Autodesk Inventor part; units mm, degrees
(part 3 of 4)
sketch "Эскиз9" plane through (0, 0, 5) normal (0, 0, 1) x (1, 0, 0)
  circle A0 centre (1.2104, 5.1192) radius 2.5 projected
  circle A1 centre (1.2104, 5.1192) radius 12.2678
  line L0 (44.0249, 7.1187) -> (57, -5.9715) projected
  line L1 (57, -5.9715) -> (57, 20.778) projected
  line L2 (53, 20.778) -> (57, 20.778) projected
  line L3 (25.3405, 9.161) -> (53, 20.778) projected
  arc A2 (16.1963, 14.3431) -> (25.3405, 9.161) centre (40.8164, 47.1281) ccw projected
  arc A3 (16.1963, 14.3431) -> (-11.1891, 14.3431) centre (2.5036, -3.8906) ccw projected
  line L4 (-11.1891, 14.3431) -> (-11.0924, 14.1698) projected
  line L5 (-11.0924, 14.1698) -> (-10.8798, 13.8428) projected
  line L6 (-10.8798, 13.8428) -> (-10.6476, 13.5415) projected
  line L7 (-10.6476, 13.5415) -> (-10.3902, 13.2744) projected
  line L8 (-10.3902, 13.2744) -> (-10.0964, 13.0589) projected
  line L9 (-10.0964, 13.0589) -> (-9.8198, 12.8188) projected
  line L10 (-9.8198, 12.8188) -> (-9.6918, 12.6838) projected
  line L11 (-9.6918, 12.6838) -> (-9.5723, 12.5363) projected
  line L12 (-9.5723, 12.5363) -> (-9.4633, 12.3731) projected
  line L13 (-9.4633, 12.3731) -> (-9.3681, 12.1883) projected
  line L14 (-9.3681, 12.1883) -> (-9.3278, 12.0845) projected
  line L15 (-9.3278, 12.0845) -> (-9.2943, 11.9695) projected
  line L16 (-9.2943, 11.9695) -> (-9.2712, 11.8376) projected
  line L17 (-9.2712, 11.8376) -> (-9.2668, 11.6743) projected
  line L18 (-9.2668, 11.6743) -> (-9.3696, 11.329) projected
  line L19 (-9.3696, 11.329) -> (-9.7265, 10.6764) projected
  line L20 (-9.7265, 10.6764) -> (-10.0432, 10.0032) projected
  line L21 (-10.0432, 10.0032) -> (-10.2615, 9.7167) projected
  line L22 (-10.2615, 9.7167) -> (-10.3959, 9.6239) projected
  line L23 (-10.3959, 9.6239) -> (-10.5161, 9.5649) projected
  line L24 (-10.5161, 9.5649) -> (-10.6287, 9.5241) projected
  line L25 (-10.6287, 9.5241) -> (-10.7364, 9.4955) projected
  line L26 (-10.7364, 9.4955) -> (-10.9417, 9.4634) projected
  line L27 (-10.9417, 9.4634) -> (-11.1379, 9.4552) projected
  line L28 (-11.1379, 9.4552) -> (-11.3274, 9.4648) projected
  line L29 (-11.3274, 9.4648) -> (-11.5119, 9.4885) projected
  line L30 (-11.5119, 9.4885) -> (-11.8689, 9.5704) projected
  line L31 (-11.8689, 9.5704) -> (-12.2162, 9.6807) projected
  line L32 (-12.2162, 9.6807) -> (-12.5837, 9.731) projected
  line L33 (-12.5837, 9.731) -> (-12.964, 9.741) projected
  line L34 (-12.964, 9.741) -> (-13.3534, 9.7199) projected
  line L35 (-13.3534, 9.7199) -> (-13.7498, 9.6714) projected
  line L36 (-13.7498, 9.6714) -> (-14.1519, 9.5976) projected
  line L37 (-14.1519, 9.5976) -> (-14.5586, 9.4998) projected
  line L38 (-14.5586, 9.4998) -> (-14.9687, 9.3787) projected
  line L39 (-14.9687, 9.3787) -> (-15.3815, 9.2349) projected
  line L40 (-15.3815, 9.2349) -> (-15.796, 9.069) projected
  line L41 (-15.796, 9.069) -> (-16.1075, 8.9301) projected
  line L42 (-16.1075, 8.9301) -> (-16.4414, 6.8067) projected
  line L43 (-16.4414, 6.8067) -> (-16.1875, 6.579) projected
  line L44 (-16.1875, 6.579) -> (-15.8439, 6.2938) projected
  line L45 (-15.8439, 6.2938) -> (-15.4952, 6.0303) projected
  line L46 (-15.4952, 6.0303) -> (-15.142, 5.7892) projected
  line L47 (-15.142, 5.7892) -> (-14.785, 5.5713) projected
  line L48 (-14.785, 5.5713) -> (-14.425, 5.3776) projected
  line L49 (-14.425, 5.3776) -> (-14.0625, 5.2099) projected
  line L50 (-14.0625, 5.2099) -> (-13.6984, 5.0703) projected
  line L51 (-13.6984, 5.0703) -> (-13.3334, 4.963) projected
  line L52 (-13.3334, 4.963) -> (-12.9682, 4.8982) projected
  line L53 (-12.9682, 4.8982) -> (-12.6038, 4.8965) projected
  line L54 (-12.6038, 4.8965) -> (-12.2389, 4.8649) projected
  line L55 (-12.2389, 4.8649) -> (-12.056, 4.8309) projected
  line L56 (-12.056, 4.8309) -> (-11.8727, 4.7818) projected
  line L57 (-11.8727, 4.7818) -> (-11.6885, 4.7139) projected
  line L58 (-11.6885, 4.7139) -> (-11.5029, 4.6203) projected
  line L59 (-11.5029, 4.6203) -> (-11.4093, 4.56) projected
  line L60 (-11.4093, 4.56) -> (-11.3146, 4.4866) projected
  line L61 (-11.3146, 4.4866) -> (-11.2183, 4.3936) projected
  line L62 (-11.2183, 4.3936) -> (-11.1188, 4.264) projected
  line L63 (-11.1188, 4.264) -> (-10.999, 3.9243) projected
  line L64 (-10.999, 3.9243) -> (-10.9042, 3.1865) projected
  line L65 (-10.9042, 3.1865) -> (-10.7647, 2.4558) projected
  line L66 (-10.7647, 2.4558) -> (-10.7729, 2.0956) projected
  line L67 (-10.7729, 2.0956) -> (-10.8272, 1.9416) projected
  line L68 (-10.8272, 1.9416) -> (-10.8897, 1.8232) projected
  line L69 (-10.8897, 1.8232) -> (-10.9568, 1.724) projected
  line L70 (-10.9568, 1.724) -> (-11.0271, 1.6375) projected
  line L71 (-11.0271, 1.6375) -> (-11.1743, 1.4909) projected
  line L72 (-11.1743, 1.4909) -> (-11.3282, 1.369) projected
  line L73 (-11.3282, 1.369) -> (-11.4872, 1.2653) projected
  line L74 (-11.4872, 1.2653) -> (-11.6504, 1.1761) projected
  line L75 (-11.6504, 1.1761) -> (-11.9874, 1.0325) projected
  line L76 (-11.9874, 1.0325) -> (-12.3332, 0.9175) projected
  line L77 (-12.3332, 0.9175) -> (-12.66, 0.7423) projected
  line L78 (-12.66, 0.7423) -> (-12.9736, 0.5268) projected
  line L79 (-12.9736, 0.5268) -> (-13.2762, 0.2808) projected
  line L80 (-13.2762, 0.2808) -> (-13.5684, 0.0086) projected
  line L81 (-13.5684, 0.0086) -> (-13.8504, -0.2874) projected
  line L82 (-13.8504, -0.2874) -> (-14.1218, -0.6056) projected
  line L83 (-14.1218, -0.6056) -> (-14.3824, -0.9447) projected
  line L84 (-14.3824, -0.9447) -> (-14.6319, -1.3036) projected
  line L85 (-14.6319, -1.3036) -> (-14.8697, -1.6815) projected
  line L86 (-14.8697, -1.6815) -> (-15.0401, -1.9769) projected
  line L87 (-15.0401, -1.9769) -> (-14.0621, -3.891) projected
  line L88 (-14.0621, -3.891) -> (-13.7228, -3.9261) projected
  line L89 (-13.7228, -3.9261) -> (-13.2773, -3.9548) projected
  line L90 (-13.2773, -3.9548) -> (-12.8403, -3.963) projected
  line L91 (-12.8403, -3.963) -> (-12.4128, -3.9505) projected
  line L92 (-12.4128, -3.9505) -> (-11.9959, -3.917) projected
  line L93 (-11.9959, -3.917) -> (-11.5908, -3.862) projected
  line L94 (-11.5908, -3.862) -> (-11.199, -3.7847) projected
  line L95 (-11.199, -3.7847) -> (-10.8224, -3.6836) projected
  line L96 (-10.8224, -3.6836) -> (-10.464, -3.5558) projected
  line L97 (-10.464, -3.5558) -> (-10.1304, -3.3936) projected
  line L98 (-10.1304, -3.3936) -> (-9.8347, -3.1808) projected
  line L99 (-9.8347, -3.1808) -> (-9.5209, -2.9918) projected
  line L100 (-9.5209, -2.9918) -> (-9.353, -2.9118) projected
  line L101 (-9.353, -2.9118) -> (-9.1758, -2.8438) projected
  line L102 (-9.1758, -2.8438) -> (-8.9868, -2.7905) projected
  line L103 (-8.9868, -2.7905) -> (-8.7817, -2.7571) projected
  line L104 (-8.7817, -2.7571) -> (-8.6705, -2.7509) projected
  line L105 (-8.6705, -2.7509) -> (-8.5508, -2.7546) projected
  line L106 (-8.5508, -2.7546) -> (-8.4182, -2.7733) projected
  line L107 (-8.4182, -2.7733) -> (-8.2615, -2.8196) projected
  line L108 (-8.2615, -2.8196) -> (-7.9649, -3.024) projected
  line L109 (-7.9649, -3.024) -> (-7.4545, -3.5652) projected
  line L110 (-7.4545, -3.5652) -> (-6.9122, -4.0744) projected
  line L111 (-6.9122, -4.0744) -> (-6.7071, -4.3705) projected
  line L112 (-6.7071, -4.3705) -> (-6.6604, -4.5271) projected
  line L113 (-6.6604, -4.5271) -> (-6.6415, -4.6596) projected
  line L114 (-6.6415, -4.6596) -> (-6.6374, -4.7793) projected
  line L115 (-6.6374, -4.7793) -> (-6.6435, -4.8906) projected
  line L116 (-6.6435, -4.8906) -> (-6.6764, -5.0958) projected
  line L117 (-6.6764, -5.0958) -> (-6.7292, -5.2848) projected
  line L118 (-6.7292, -5.2848) -> (-6.7969, -5.4622) projected
  line L119 (-6.7969, -5.4622) -> (-6.8765, -5.6303) projected
  line L120 (-6.8765, -5.6303) -> (-7.0647, -5.9445) projected
  line L121 (-7.0647, -5.9445) -> (-7.2769, -6.2407) projected
  line L122 (-7.2769, -6.2407) -> (-7.4384, -6.5746) projected
  line L123 (-7.4384, -6.5746) -> (-7.5654, -6.9333) projected
  line L124 (-7.5654, -6.9333) -> (-7.6656, -7.3102) projected
  line L125 (-7.6656, -7.3102) -> (-7.742, -7.7022) projected
  line L126 (-7.742, -7.7022) -> (-7.7961, -8.1074) projected
  line L127 (-7.7961, -8.1074) -> (-7.8287, -8.5243) projected
  line L128 (-7.8287, -8.5243) -> (-7.8403, -8.9518) projected
  line L129 (-7.8403, -8.9518) -> (-7.8311, -9.3888) projected
  line L130 (-7.8311, -9.3888) -> (-7.8013, -9.8343) projected
  line L131 (-7.8013, -9.8343) -> (-7.7656, -10.1735) projected
  line L132 (-7.7656, -10.1735) -> (-5.8492, -11.1472) projected
  line L133 (-5.8492, -11.1472) -> (-5.5542, -10.9761) projected
  line L134 (-5.5542, -10.9761) -> (-5.1768, -10.7375) projected
  line L135 (-5.1768, -10.7375) -> (-4.8185, -10.4872) projected
  line L136 (-4.8185, -10.4872) -> (-4.48, -10.2258) projected
  line L137 (-4.48, -10.2258) -> (-4.1624, -9.9537) projected
  line L138 (-4.1624, -9.9537) -> (-3.867, -9.6711) projected
  line L139 (-3.867, -9.6711) -> (-3.5955, -9.3782) projected
  line L140 (-3.5955, -9.3782) -> (-3.3502, -9.0751) projected
  line L141 (-3.3502, -9.0751) -> (-3.1354, -8.7611) projected
  line L142 (-3.1354, -8.7611) -> (-2.9609, -8.4338) projected
  line L143 (-2.9609, -8.4338) -> (-2.8467, -8.0877) projected
  line L144 (-2.8467, -8.0877) -> (-2.7039, -7.7505) projected
  line L145 (-2.7039, -7.7505) -> (-2.615, -7.5871) projected
  line L146 (-2.615, -7.5871) -> (-2.5117, -7.4278) projected
  line L147 (-2.5117, -7.4278) -> (-2.3901, -7.2737) projected
  line L148 (-2.3901, -7.2737) -> (-2.2438, -7.1261) projected
  line L149 (-2.2438, -7.1261) -> (-2.1575, -7.0556) projected
  line L150 (-2.1575, -7.0556) -> (-2.0585, -6.9883) projected
  line L151 (-2.0585, -6.9883) -> (-1.9402, -6.9255) projected
  line L152 (-1.9402, -6.9255) -> (-1.7863, -6.8709) projected
  line L153 (-1.7863, -6.8709) -> (-1.4262, -6.8619) projected
  line L154 (-1.4262, -6.8619) -> (-0.6951, -6.9997) projected
  line L155 (-0.6951, -6.9997) -> (0.0429, -7.0929) projected
  line L156 (0.0429, -7.0929) -> (0.3829, -7.2119) projected
  line L157 (0.3829, -7.2119) -> (0.5127, -7.3112) projected
  line L158 (0.5127, -7.3112) -> (0.6059, -7.4072) projected
  line L159 (0.6059, -7.4072) -> (0.6795, -7.5017) projected
  line L160 (0.6795, -7.5017) -> (0.74, -7.5953) projected
  line L161 (0.74, -7.5953) -> (0.834, -7.7806) projected
  line L162 (0.834, -7.7806) -> (0.9024, -7.9646) projected
  line L163 (0.9024, -7.9646) -> (0.9519, -8.1479) projected
  line L164 (0.9519, -8.1479) -> (0.9863, -8.3307) projected
  line L165 (0.9863, -8.3307) -> (1.0187, -8.6955) projected
  line L166 (1.0187, -8.6955) -> (1.0212, -9.0599) projected
  line L167 (1.0212, -9.0599) -> (1.0869, -9.4249) projected
  line L168 (1.0869, -9.4249) -> (1.1949, -9.7897) projected
  line L169 (1.1949, -9.7897) -> (1.3353, -10.1535) projected
  line L170 (1.3353, -10.1535) -> (1.5039, -10.5156) projected
  line L171 (1.5039, -10.5156) -> (1.6983, -10.8752) projected
  line L172 (1.6983, -10.8752) -> (1.9171, -11.2317) projected
  line L173 (1.9171, -11.2317) -> (2.159, -11.5843) projected
  line L174 (2.159, -11.5843) -> (2.4233, -11.9325) projected
  line L175 (2.4233, -11.9325) -> (2.7092, -12.2754) projected
  line L176 (2.7092, -12.2754) -> (2.9375, -12.5288) projected
  line L177 (2.9375, -12.5288) -> (5.0602, -12.1901) projected
  line L178 (5.0602, -12.1901) -> (5.1983, -11.8783) projected
  line L179 (5.1983, -11.8783) -> (5.3633, -11.4634) projected
  line L180 (5.3633, -11.4634) -> (5.5062, -11.0504) projected
  line L181 (5.5062, -11.0504) -> (5.6263, -10.6399) projected
  line L182 (5.6263, -10.6399) -> (5.7233, -10.2331) projected
  line L183 (5.7233, -10.2331) -> (5.7962, -9.8308) projected
  line L184 (5.7962, -9.8308) -> (5.8437, -9.4343) projected
  line L185 (5.8437, -9.4343) -> (5.864, -9.0449) projected
  line L186 (5.864, -9.0449) -> (5.8532, -8.6645) projected
  line L187 (5.8532, -8.6645) -> (5.802, -8.2972) projected
  line L188 (5.802, -8.2972) -> (5.691, -7.9502) projected
  line L189 (5.691, -7.9502) -> (5.6083, -7.5933) projected
  line L190 (5.6083, -7.5933) -> (5.5841, -7.4089) projected
  line L191 (5.5841, -7.4089) -> (5.5741, -7.2193) projected
  line L192 (5.5741, -7.2193) -> (5.5818, -7.0232) projected
  line L193 (5.5818, -7.0232) -> (5.6135, -6.8178) projected
  line L194 (5.6135, -6.8178) -> (5.6419, -6.7101) projected
  line L195 (5.6419, -6.7101) -> (5.6824, -6.5974) projected
  line L196 (5.6824, -6.5974) -> (5.7412, -6.4771) projected
  line L197 (5.7412, -6.4771) -> (5.8336, -6.3424) projected
  line L198 (5.8336, -6.3424) -> (6.1197, -6.1235) projected
  line L199 (6.1197, -6.1235) -> (6.7921, -5.8052) projected
  line L200 (6.7921, -5.8052) -> (7.444, -5.4468) projected
  line L201 (7.444, -5.4468) -> (7.789, -5.3433) projected
  line L202 (7.789, -5.3433) -> (7.9523, -5.3473) projected
  line L203 (7.9523, -5.3473) -> (8.0842, -5.3702) projected
  line L204 (8.0842, -5.3702) -> (25.3405, 4.0009) projected
  line L205 (40.9018, 10.5367) -> (25.3405, 4.0009) projected
  line L206 (40.9018, 10.5367) -> (44.0249, 7.1187) projected
  circle A4 centre (1.2104, 5.1192) radius 2.5 projected
  circle A5 centre (4.7663, 12.2855) radius 1.6 projected
  circle A6 centre (-5.9559, 8.675) radius 1.6 projected
  circle A7 centre (-2.3455, -2.0471) radius 1.6 projected
  circle A8 centre (8.3767, 1.5633) radius 1.6 projected
  point P0 (0, 0)
  point P1 (-10.9042, 3.1865)
  constraints: 1 coincident, 3 other
extrude "Выдавливание9" cut sketch "Эскиз9" against normal through all contours A1 L18 L17 L16 L15 L14 L13 L12 L11 L10 L9 L8 L7 L6 L5 L4 A3 A2 L3 L2 L1 L0 L206 L205 L204 L203 L202 L201
sketch "Эскиз18" plane through (0, 0, 5) normal (0, 0, 1) x (1, 0, 0)
  arc A0 (-3.5282, 16.5591) -> (-4.3322, 16.1919) centre (1.2104, 5.1192) ccw
  arc A1 (-6.5592, 14.7607) -> (-7.2273, 14.1819) centre (1.2104, 5.1192) ccw
  arc A2 (-8.9608, 12.1812) -> (-9.4387, 11.4376) centre (1.2104, 5.1192) ccw
  arc A3 (-10.7875, 8.1814) -> (-13.7875, 7.8251) centre (-10.997, -2.8603) ccw
  arc A4 (-13.7875, 7.8251) -> (-13.9423, 6.7483) centre (1.2104, 5.1192) ccw
  arc A5 (-13.9423, 6.7483) -> (-11.1642, 5.5611) centre (-8.2544, 16.2146) ccw
  arc A6 (-11.1642, 5.5611) -> (-11.1642, 4.6772) centre (1.2104, 5.1192) ccw
  arc A7 (-11.1642, 4.6772) -> (-13.9423, 3.4901) centre (-8.2544, -5.9763) ccw
  arc A8 (-13.9423, 3.4901) -> (-13.7875, 2.4133) centre (1.2104, 5.1192) ccw
  arc A9 (-13.7875, 2.4133) -> (-10.7875, 2.0569) centre (-10.997, 13.0986) ccw
  arc A10 (-10.7875, 2.0569) -> (-10.5384, 1.2088) centre (1.2104, 5.1192) ccw
  arc A11 (-10.5384, 1.2088) -> (-12.8695, -0.7129) centre (-4.7451, -8.1934) ccw
  arc A12 (-12.8695, -0.7129) -> (-12.4176, -1.7025) centre (1.2104, 5.1192) ccw
  arc A13 (-12.4176, -1.7025) -> (-9.4387, -1.1992) centre (-12.7506, 9.3362) ccw
  arc A14 (-9.4387, -1.1992) -> (-8.9608, -1.9429) centre (1.2104, 5.1192) ccw
  arc A15 (-8.9608, -1.9429) -> (-10.6561, -4.4435) centre (-0.7533, -9.332) ccw
  arc A16 (-10.6561, -4.4435) -> (-9.9437, -5.2656) centre (1.2104, 5.1192) ccw
  arc A17 (-9.9437, -5.2656) -> (-7.2273, -3.9435) centre (-13.3732, 5.2321) ccw
  arc A18 (-7.2273, -3.9435) -> (-6.5592, -4.5224) centre (1.2104, 5.1192) ccw
  arc A19 (-6.5592, -4.5224) -> (-7.4813, -7.3993) centre (3.3977, -9.2999) ccw
  arc A20 (-7.4813, -7.3993) -> (-6.5661, -7.9874) centre (1.2104, 5.1192) ccw
  arc A21 (-6.5661, -7.9874) -> (-4.3322, -5.9536) centre (-12.8142, 1.1189) ccw
  arc A22 (-4.3322, -5.9536) -> (-3.5282, -6.3208) centre (1.2104, 5.1192) ccw
  arc A23 (-3.5282, -6.3208) -> (-3.6024, -9.3409) centre (7.3714, -8.0996) ccw
  arc A24 (-3.6024, -9.3409) -> (-2.5586, -9.6474) centre (1.2104, 5.1192) ccw
  arc A25 (-2.5586, -9.6474) -> (-0.9882, -7.0666) centre (-11.1191, -2.6703) ccw
  arc A26 (-0.9882, -7.0666) -> (-0.1132, -7.1924) centre (1.2104, 5.1192) ccw
  arc A27 (-0.1132, -7.1924) -> (0.6664, -10.1111) centre (10.846, -5.8284) ccw
  arc A28 (0.6664, -10.1111) -> (1.7543, -10.1111) centre (1.2104, 5.1192) ccw
  arc A29 (1.7543, -10.1111) -> (2.534, -7.1924) centre (-8.4252, -5.8284) ccw
  arc A30 (2.534, -7.1924) -> (3.409, -7.0666) centre (1.2104, 5.1192) ccw
  arc A31 (3.409, -7.0666) -> (4.9793, -9.6474) centre (13.5399, -2.6703) ccw
  arc A32 (4.9793, -9.6474) -> (6.0232, -9.3409) centre (1.2104, 5.1192) ccw
  arc A33 (6.0232, -9.3409) -> (5.949, -6.3208) centre (-4.9506, -8.0996) ccw
  arc A34 (5.949, -6.3208) -> (6.753, -5.9536) centre (1.2104, 5.1192) ccw
  arc A35 (8.98, -4.5224) -> (9.6481, -3.9435) centre (1.2104, 5.1192) ccw
  arc A36 (11.3816, -1.9429) -> (11.8595, -1.1992) centre (1.2104, 5.1192) ccw
  arc A37 (12.9592, 1.2088) -> (13.2083, 2.0569) centre (1.2104, 5.1192) ccw
  arc A38 (13.585, 4.6772) -> (13.585, 5.5611) centre (1.2104, 5.1192) ccw
  arc A39 (13.2083, 8.1814) -> (12.9592, 9.0296) centre (1.2104, 5.1192) ccw
  arc A40 (11.8595, 11.4376) -> (11.3816, 12.1812) centre (1.2104, 5.1192) ccw
  arc A41 (9.6481, 14.1819) -> (8.98, 14.7607) centre (1.2104, 5.1192) ccw
  arc A42 (6.753, 16.1919) -> (5.949, 16.5591) centre (1.2104, 5.1192) ccw
  arc A43 (3.409, 17.3049) -> (2.534, 17.4307) centre (1.2104, 5.1192) ccw
  arc A44 (-0.1132, 17.4307) -> (-0.9882, 17.3049) centre (1.2104, 5.1192) ccw
  circle A45 centre (1.2104, 5.1192) radius 2.5 projected
  circle A46 centre (-2.3455, -2.0471) radius 1.6 projected
  circle A47 centre (-5.9559, 8.675) radius 1.6 projected
  circle A48 centre (8.3767, 1.5633) radius 1.6 projected
  circle A49 centre (4.7663, 12.2855) radius 1.6 projected
  circle A50 centre (1.2104, 5.1192) radius 12.3825
  line L0 (-10.7875, 8.1814) -> (1.2104, 5.1192)
  point P0 (0, 0)
  point P1 (1.2104, 5.1192)
  point P2 (6.753, -5.9536)
  point P3 (8.98, -4.5224)
  point P4 (9.6481, -3.9435)
  point P5 (11.3816, -1.9429)
  point P6 (11.8595, -1.1992)
  point P7 (13.2083, 2.0569)
  point P8 (13.585, 4.6772)
  point P9 (13.585, 5.5611)
  point P10 (13.2083, 8.1814)
  point P11 (12.9592, 9.0296)
  point P12 (11.8595, 11.4376)
  point P13 (11.3816, 12.1812)
  point P14 (8.98, 14.7607)
  point P15 (5.949, 16.5591)
  point P16 (3.409, 17.3049)
  point P17 (2.534, 17.4307)
  point P18 (-0.1132, 17.4307)
  point P19 (-0.9882, 17.3049)
  point P20 (-3.5282, 16.5591)
  point P21 (-4.3322, 16.1919)
  point P22 (-6.5592, 14.7607)
  point P23 (-7.2273, 14.1819)
  point P24 (-9.4387, 11.4376)
  point P25 (3.409, -7.0666)
  point P26 (2.534, -7.1924)
  point P27 (-0.1132, -7.1924)
  point P28 (-0.9882, -7.0666)
  point P29 (-3.5282, -6.3208)
  point P30 (-4.3322, -5.9536)
  point P31 (-6.5592, -4.5224)
  point P32 (-7.2273, -3.9435)
  point P33 (-8.9608, -1.9429)
  point P34 (-9.4387, -1.1992)
  point P35 (-10.5384, 1.2088)
  point P36 (-10.7875, 2.0569)
  point P37 (-11.1642, 4.6772)
  point P38 (-11.1642, 5.5611)
  constraints: 90 point on circle, 45 centre point, 2 end point, 1 coincident, 4 other
sketch "Эскиз19" plane through (0, 0, 5) normal (0, 0, 1) x (1, 0, 0)
  arc A0 (7.444, -5.4468) -> (-9.3696, 11.329) centre (1.2104, 5.1192) ccw projected
  line L0 (-9.3696, 11.329) -> (-9.7265, 10.6764) projected
  line L1 (-9.7265, 10.6764) -> (-10.0432, 10.0032) projected
  line L2 (-10.0432, 10.0032) -> (-10.2615, 9.7167) projected
  line L3 (-10.2615, 9.7167) -> (-10.3959, 9.6239) projected
  line L4 (-10.3959, 9.6239) -> (-10.5161, 9.5649) projected
  line L5 (-10.5161, 9.5649) -> (-10.6287, 9.5241) projected
  line L6 (-10.6287, 9.5241) -> (-10.7364, 9.4955) projected
  line L7 (-10.7364, 9.4955) -> (-10.9417, 9.4634) projected
  line L8 (-10.9417, 9.4634) -> (-11.1379, 9.4552) projected
  line L9 (-11.1379, 9.4552) -> (-11.3274, 9.4648) projected
  line L10 (-11.3274, 9.4648) -> (-11.5119, 9.4885) projected
  line L11 (-11.5119, 9.4885) -> (-11.8689, 9.5704) projected
  line L12 (-11.8689, 9.5704) -> (-12.2162, 9.6807) projected
  line L13 (-12.2162, 9.6807) -> (-12.5837, 9.731) projected
  line L14 (-12.5837, 9.731) -> (-12.964, 9.741) projected
  line L15 (-12.964, 9.741) -> (-13.3534, 9.7199) projected
  line L16 (-13.3534, 9.7199) -> (-13.7498, 9.6714) projected
  line L17 (-13.7498, 9.6714) -> (-14.1519, 9.5976) projected
  line L18 (-14.1519, 9.5976) -> (-14.5586, 9.4998) projected
  line L19 (-14.5586, 9.4998) -> (-14.9687, 9.3787) projected
  line L20 (-14.9687, 9.3787) -> (-15.3815, 9.2349) projected
  line L21 (-15.3815, 9.2349) -> (-15.796, 9.069) projected
  line L22 (-15.796, 9.069) -> (-16.1075, 8.9301) projected
  line L23 (-16.1075, 8.9301) -> (-16.4414, 6.8067) projected
  line L24 (-16.4414, 6.8067) -> (-16.1875, 6.579) projected
  line L25 (-16.1875, 6.579) -> (-15.8439, 6.2938) projected
  line L26 (-15.8439, 6.2938) -> (-15.4952, 6.0303) projected
  line L27 (-15.4952, 6.0303) -> (-15.142, 5.7892) projected
  line L28 (-15.142, 5.7892) -> (-14.785, 5.5713) projected
  line L29 (-14.785, 5.5713) -> (-14.425, 5.3776) projected
  line L30 (-14.425, 5.3776) -> (-14.0625, 5.2099) projected
  line L31 (-14.0625, 5.2099) -> (-13.6984, 5.0703) projected
  line L32 (-13.6984, 5.0703) -> (-13.3334, 4.963) projected
  line L33 (-13.3334, 4.963) -> (-12.9682, 4.8982) projected
  line L34 (-12.9682, 4.8982) -> (-12.6038, 4.8965) projected
  line L35 (-12.6038, 4.8965) -> (-12.2389, 4.8649) projected
  line L36 (-12.2389, 4.8649) -> (-12.056, 4.8309) projected
  line L37 (-12.056, 4.8309) -> (-11.8727, 4.7818) projected
  line L38 (-11.8727, 4.7818) -> (-11.6885, 4.7139) projected
  line L39 (-11.6885, 4.7139) -> (-11.5029, 4.6203) projected
  line L40 (-11.5029, 4.6203) -> (-11.4093, 4.56) projected
  line L41 (-11.4093, 4.56) -> (-11.3146, 4.4866) projected
  line L42 (-11.3146, 4.4866) -> (-11.2183, 4.3936) projected
  line L43 (-11.2183, 4.3936) -> (-11.1188, 4.264) projected
  line L44 (-11.1188, 4.264) -> (-10.999, 3.9243) projected
  line L45 (-10.999, 3.9243) -> (-10.9042, 3.1865) projected
  line L46 (-10.9042, 3.1865) -> (-10.7647, 2.4558) projected
  line L47 (-10.7647, 2.4558) -> (-10.7729, 2.0956) projected
  line L48 (-10.7729, 2.0956) -> (-10.8272, 1.9416) projected
  line L49 (-10.8272, 1.9416) -> (-10.8897, 1.8232) projected
  line L50 (-10.8897, 1.8232) -> (-10.9568, 1.724) projected
  line L51 (-10.9568, 1.724) -> (-11.0271, 1.6375) projected
  line L52 (-11.0271, 1.6375) -> (-11.1743, 1.4909) projected
  line L53 (-11.1743, 1.4909) -> (-11.3282, 1.369) projected
  line L54 (-11.3282, 1.369) -> (-11.4872, 1.2653) projected
  line L55 (-11.4872, 1.2653) -> (-11.6504, 1.1761) projected
  line L56 (-11.6504, 1.1761) -> (-11.9874, 1.0325) projected
  line L57 (-11.9874, 1.0325) -> (-12.3332, 0.9175) projected
  line L58 (-12.3332, 0.9175) -> (-12.66, 0.7423) projected
  line L59 (-12.66, 0.7423) -> (-12.9736, 0.5268) projected
  line L60 (-12.9736, 0.5268) -> (-13.2762, 0.2808) projected
  line L61 (-13.2762, 0.2808) -> (-13.5684, 0.0086) projected
  line L62 (-13.5684, 0.0086) -> (-13.8504, -0.2874) projected
  line L63 (-13.8504, -0.2874) -> (-14.1218, -0.6056) projected
  line L64 (-14.1218, -0.6056) -> (-14.3824, -0.9447) projected
  line L65 (-14.3824, -0.9447) -> (-14.6319, -1.3036) projected
  line L66 (-14.6319, -1.3036) -> (-14.8697, -1.6815) projected
  line L67 (-14.8697, -1.6815) -> (-15.0401, -1.9769) projected
  line L68 (-15.0401, -1.9769) -> (-14.0621, -3.891) projected
  line L69 (-14.0621, -3.891) -> (-13.7228, -3.9261) projected
  line L70 (-13.7228, -3.9261) -> (-13.2773, -3.9548) projected
  line L71 (-13.2773, -3.9548) -> (-12.8403, -3.963) projected
  line L72 (-12.8403, -3.963) -> (-12.4128, -3.9505) projected
  line L73 (-12.4128, -3.9505) -> (-11.9959, -3.917) projected
  line L74 (-11.9959, -3.917) -> (-11.5908, -3.862) projected
  line L75 (-11.5908, -3.862) -> (-11.199, -3.7847) projected
  line L76 (-11.199, -3.7847) -> (-10.8224, -3.6836) projected
  line L77 (-10.8224, -3.6836) -> (-10.464, -3.5558) projected
  line L78 (-10.464, -3.5558) -> (-10.1304, -3.3936) projected
  line L79 (-10.1304, -3.3936) -> (-9.8347, -3.1808) projected
  line L80 (-9.8347, -3.1808) -> (-9.5209, -2.9918) projected
  line L81 (-9.5209, -2.9918) -> (-9.353, -2.9118) projected
  line L82 (-9.353, -2.9118) -> (-9.1758, -2.8438) projected
  line L83 (-9.1758, -2.8438) -> (-8.9868, -2.7905) projected
  line L84 (-8.9868, -2.7905) -> (-8.7817, -2.7571) projected
  line L85 (-8.7817, -2.7571) -> (-8.6705, -2.7509) projected
  line L86 (-8.6705, -2.7509) -> (-8.5508, -2.7546) projected
  line L87 (-8.5508, -2.7546) -> (-8.4182, -2.7733) projected
  line L88 (-8.4182, -2.7733) -> (-8.2615, -2.8196) projected
  line L89 (-8.2615, -2.8196) -> (-7.9649, -3.024) projected
  line L90 (-7.9649, -3.024) -> (-7.4545, -3.5652) projected
  line L91 (-7.4545, -3.5652) -> (-6.9122, -4.0744) projected
  line L92 (-6.9122, -4.0744) -> (-6.7071, -4.3705) projected
  line L93 (-6.7071, -4.3705) -> (-6.6604, -4.5271) projected
  line L94 (-6.6604, -4.5271) -> (-6.6415, -4.6596) projected
  line L95 (-6.6415, -4.6596) -> (-6.6374, -4.7793) projected
  line L96 (-6.6374, -4.7793) -> (-6.6435, -4.8906) projected
  line L97 (-6.6435, -4.8906) -> (-6.6764, -5.0958) projected
  line L98 (-6.6764, -5.0958) -> (-6.7292, -5.2848) projected
  line L99 (-6.7292, -5.2848) -> (-6.7969, -5.4622) projected
  line L100 (-6.7969, -5.4622) -> (-6.8765, -5.6303) projected
  line L101 (-6.8765, -5.6303) -> (-7.0647, -5.9445) projected
  line L102 (-7.0647, -5.9445) -> (-7.2769, -6.2407) projected
  line L103 (-7.2769, -6.2407) -> (-7.4384, -6.5746) projected
  line L104 (-7.4384, -6.5746) -> (-7.5654, -6.9333) projected
  line L105 (-7.5654, -6.9333) -> (-7.6656, -7.3102) projected
  line L106 (-7.6656, -7.3102) -> (-7.742, -7.7022) projected
  line L107 (-7.742, -7.7022) -> (-7.7961, -8.1074) projected
  line L108 (-7.7961, -8.1074) -> (-7.8287, -8.5243) projected
  line L109 (-7.8287, -8.5243) -> (-7.8403, -8.9518) projected
  line L110 (-7.8403, -8.9518) -> (-7.8311, -9.3888) projected
  line L111 (-7.8311, -9.3888) -> (-7.8013, -9.8343) projected
  line L112 (-7.8013, -9.8343) -> (-7.7656, -10.1735) projected
  line L113 (-7.7656, -10.1735) -> (-5.8492, -11.1472) projected
  line L114 (-5.8492, -11.1472) -> (-5.5542, -10.9761) projected
  line L115 (-5.5542, -10.9761) -> (-5.1768, -10.7375) projected
  line L116 (-5.1768, -10.7375) -> (-4.8185, -10.4872) projected
  line L117 (-4.8185, -10.4872) -> (-4.48, -10.2258) projected
  line L118 (-4.48, -10.2258) -> (-4.1624, -9.9537) projected
  line L119 (-4.1624, -9.9537) -> (-3.867, -9.6711) projected
  line L120 (-3.867, -9.6711) -> (-3.5955, -9.3782) projected
  line L121 (-3.5955, -9.3782) -> (-3.3502, -9.0751) projected
  line L122 (-3.3502, -9.0751) -> (-3.1354, -8.7611) projected
  line L123 (-3.1354, -8.7611) -> (-2.9609, -8.4338) projected
  line L124 (-2.9609, -8.4338) -> (-2.8467, -8.0877) projected
  line L125 (-2.8467, -8.0877) -> (-2.7039, -7.7505) projected
  line L126 (-2.7039, -7.7505) -> (-2.615, -7.5871) projected
  line L127 (-2.615, -7.5871) -> (-2.5117, -7.4278) projected
  line L128 (-2.5117, -7.4278) -> (-2.3901, -7.2737) projected
  line L129 (-2.3901, -7.2737) -> (-2.2438, -7.1261) projected
  line L130 (-2.2438, -7.1261) -> (-2.1575, -7.0556) projected
  line L131 (-2.1575, -7.0556) -> (-2.0585, -6.9883) projected
  line L132 (-2.0585, -6.9883) -> (-1.9402, -6.9255) projected
  line L133 (-1.9402, -6.9255) -> (-1.7863, -6.8709) projected
  line L134 (-1.7863, -6.8709) -> (-1.4262, -6.8619) projected
  line L135 (-1.4262, -6.8619) -> (-0.6951, -6.9997) projected
  line L136 (-0.6951, -6.9997) -> (0.0429, -7.0929) projected
  line L137 (0.0429, -7.0929) -> (0.3829, -7.2119) projected
  line L138 (0.3829, -7.2119) -> (0.5127, -7.3112) projected
  line L139 (0.5127, -7.3112) -> (0.6059, -7.4072) projected
  line L140 (0.6059, -7.4072) -> (0.6795, -7.5017) projected
  line L141 (0.6795, -7.5017) -> (0.74, -7.5953) projected
  line L142 (0.74, -7.5953) -> (0.834, -7.7806) projected
  line L143 (0.834, -7.7806) -> (0.9024, -7.9646) projected
  line L144 (0.9024, -7.9646) -> (0.9519, -8.1479) projected
  line L145 (0.9519, -8.1479) -> (0.9863, -8.3307) projected
  line L146 (0.9863, -8.3307) -> (1.0187, -8.6955) projected
  line L147 (1.0187, -8.6955) -> (1.0212, -9.0599) projected
  line L148 (1.0212, -9.0599) -> (1.0869, -9.4249) projected
  line L149 (1.0869, -9.4249) -> (1.1949, -9.7897) projected
  line L150 (1.1949, -9.7897) -> (1.3353, -10.1535) projected
  line L151 (1.3353, -10.1535) -> (1.5039, -10.5156) projected
  line L152 (1.5039, -10.5156) -> (1.6983, -10.8752) projected
  line L153 (1.6983, -10.8752) -> (1.9171, -11.2317) projected
  line L154 (1.9171, -11.2317) -> (2.159, -11.5843) projected
  line L155 (2.159, -11.5843) -> (2.4233, -11.9325) projected
  line L156 (2.4233, -11.9325) -> (2.7092, -12.2754) projected
  line L157 (2.7092, -12.2754) -> (2.9375, -12.5288) projected
  line L158 (2.9375, -12.5288) -> (5.0602, -12.1901) projected
  line L159 (5.0602, -12.1901) -> (5.1983, -11.8783) projected
  line L160 (5.1983, -11.8783) -> (5.3633, -11.4634) projected
  line L161 (5.3633, -11.4634) -> (5.5062, -11.0504) projected
  line L162 (5.5062, -11.0504) -> (5.6263, -10.6399) projected
  line L163 (5.6263, -10.6399) -> (5.7233, -10.2331) projected
  line L164 (5.7233, -10.2331) -> (5.7962, -9.8308) projected
  line L165 (5.7962, -9.8308) -> (5.8437, -9.4343) projected
  line L166 (5.8437, -9.4343) -> (5.864, -9.0449) projected
  line L167 (5.864, -9.0449) -> (5.8532, -8.6645) projected
  line L168 (5.8532, -8.6645) -> (5.802, -8.2972) projected
  line L169 (5.802, -8.2972) -> (5.691, -7.9502) projected
  line L170 (5.691, -7.9502) -> (5.6083, -7.5933) projected
  line L171 (5.6083, -7.5933) -> (5.5841, -7.4089) projected
  line L172 (5.5841, -7.4089) -> (5.5741, -7.2193) projected
  line L173 (5.5741, -7.2193) -> (5.5818, -7.0232) projected
  line L174 (5.5818, -7.0232) -> (5.6135, -6.8178) projected
  line L175 (5.6135, -6.8178) -> (5.6419, -6.7101) projected
  line L176 (5.6419, -6.7101) -> (5.6824, -6.5974) projected
  line L177 (5.6824, -6.5974) -> (5.7412, -6.4771) projected
  line L178 (5.7412, -6.4771) -> (5.8336, -6.3424) projected
  line L179 (5.8336, -6.3424) -> (6.1197, -6.1235) projected
  line L180 (6.1197, -6.1235) -> (6.7921, -5.8052) projected
  line L181 (6.7921, -5.8052) -> (7.444, -5.4468) projected
  circle A1 centre (1.2104, 5.1192) radius 2.5 projected
  circle A2 centre (4.7663, 12.2855) radius 1.6 projected
  circle A3 centre (-5.9559, 8.675) radius 1.6 projected
  circle A4 centre (-2.3455, -2.0471) radius 1.6 projected
  circle A5 centre (8.3767, 1.5633) radius 1.6 projected
  circle A6 centre (1.2104, 5.1192) radius 12.2678
  point P0 (0, 0)
  point P1 (0.0425, -7.0929)
  constraints: 1 centre point, 1 coincident, 1 concentric
extrude "Выдавливание17" cut sketch "Эскиз19" against normal blind 10 contours L179 L178 L177 L176 L175 L174 L173 L172 L171 L170 L169 L168 L167 L166 L165 L164 L163 L162 L161 L160 L159 L158 L157 L156 L155 L154 L153 L152 L151 L150 L149 L148 L147 L146 L145 L144 L143 L142 L141 L140 L139 L138 L137 A6 | A6 L44 L43 L42 L41 L40 L39 L38 L37 L36 L35 L34 L33 L32 L31 L30 L29 L28 L27 L26 L25 L24 L23 L22 L21 L20 L19 L18 L17 L16 L15 L14 L13 L12 L11 L10 L9 L8 L7 L6 L5 L4 L3 L2 | L134 L133 L132 L131 L130 L129 L128 L127 L126 L125 L124 L123 L122 L121 L120 L119 L118 L117 L116 L115 L114 L113 L112 L111 L110 L109 L108 L107 L106 L105 L104 L103 L102 L101 L100 L99 L98 L97 L96 L95 L94 L93 L92 A6 | A6 L89 L88 L87 L86 L85 L84 L83 L82 L81 L80 L79 L78 L77 L76 L75 L74 L73 L72 L71 L70 L69 L68 L67 L66 L65 L64 L63 L62 L61 L60 L59 L58 L57 L56 L55 L54 L53 L52 L51 L50 L49 L48 L47
extrude "Выдавливание19" add sketch "Эскиз18" against normal up to surface (5 mm away)
sketch "Эскиз20" plane through (0, 0, 5) normal (0, 0, 1) x (1, 0, 0)
  point P0 (0, 0)
sketch "Эскиз22" plane through (0, 0, 5) normal (0, 0, 1) x (1, 0, 0)
  arc A0 (-16.2957, -2.2293) -> (-17.3109, -5.0747) centre (-6.4996, -7.3285) ccw projected
  arc A1 (-17.3109, -5.0747) -> (-18.1932, -5.1286) centre (-16.9965, -17.4532) ccw projected
  arc A2 (-18.1932, -5.1286) -> (-19.5478, -2.4282) centre (-28.6492, -8.6835) ccw projected
  arc A3 (-19.5478, -2.4282) -> (-20.6131, -2.6485) centre (-16.9965, -17.4532) ccw projected
  arc A4 (-20.6131, -2.6485) -> (-20.7856, -5.6647) centre (-9.7773, -4.7813) ccw projected
  arc A5 (-20.7856, -5.6647) -> (-25.7458, -8.691) centre (-16.9965, -17.4532) ccw projected
  line L0 (-43.1204, -4.145) -> (-44.248, -1.3649) projected
  line L1 (-46.546, 18.0729) -> (-53.6271, 17.2356) projected
  line L2 (-53.6271, 17.2356) -> (-50.9363, -5.5221) projected
  line L3 (-50.9363, -5.5221) -> (-49.1028, -10.0428) projected
  arc A6 (-25.2458, -26.6876) -> (-5.2885, -21.4844) centre (-16.9965, -17.4532) ccw projected
  arc A7 (-5.2885, -21.4844) -> (-2.2695, -21.374) centre (-4.1786, -10.4965) ccw projected
  arc A8 (-2.2695, -21.374) -> (-2.0273, -20.3134) centre (-16.9965, -17.4532) ccw projected
  arc A9 (-2.0273, -20.3134) -> (-4.6992, -18.9035) centre (-8.4687, -29.284) ccw projected
  arc A10 (-4.6992, -18.9035) -> (-4.6271, -18.0226) centre (-16.9965, -17.4532) ccw projected
  arc A11 (-4.6271, -18.0226) -> (-1.7614, -17.0661) centre (-6.6577, -7.1671) ccw projected
  arc A12 (-1.7614, -17.0661) -> (-1.8278, -15.9802) centre (-16.9965, -17.4532) ccw projected
  arc A13 (-1.8278, -15.9802) -> (-4.7887, -15.3802) centre (-5.481, -26.4023) ccw projected
  arc A14 (-4.7887, -15.3802) -> (-4.9677, -14.5146) centre (-16.9965, -17.4532) ccw projected
  arc A15 (-4.9677, -14.5146) -> (-2.4876, -12.7896) centre (-9.9744, -4.671) ccw projected
  arc A16 (-2.4876, -12.7896) -> (-2.8572, -11.7664) centre (-16.9965, -17.4532) ccw projected
  arc A17 (-2.8572, -11.7664) -> (-5.8672, -12.0249) centre (-3.4262, -22.7955) ccw projected
  arc A18 (-5.8672, -12.0249) -> (-6.2828, -11.2448) centre (-16.9965, -17.4532) ccw projected
  arc A19 (-6.2828, -11.2448) -> (-4.3892, -8.8908) centre (-13.86, -3.2104) ccw projected
  arc A20 (-4.3892, -8.8908) -> (-5.0321, -8.0133) centre (-16.9965, -17.4532) ccw projected
  arc A21 (-5.0321, -8.0133) -> (-7.8474, -9.1093) centre (-2.4708, -18.7559) ccw projected
  arc A22 (-7.8474, -9.1093) -> (-8.4659, -8.4779) centre (-16.9965, -17.4532) ccw projected
  arc A23 (-8.4659, -8.4779) -> (-7.3121, -5.6858) centre (-17.9997, -2.9037) ccw projected
  arc A24 (-7.3121, -5.6858) -> (-8.1763, -5.0249) centre (-16.9965, -17.4532) ccw projected
  arc A25 (-8.1763, -5.0249) -> (-10.5687, -6.8697) centre (-2.6921, -14.6107) ccw projected
  arc A26 (-10.5687, -6.8697) -> (-11.3401, -6.4381) centre (-16.9965, -17.4532) ccw projected
  arc A27 (-11.3401, -6.4381) -> (-11.0197, -3.4341) centre (-22.0581, -3.7757) ccw projected
  arc A28 (-11.0197, -3.4341) -> (-12.035, -3.0434) centre (-16.9965, -17.4532) ccw projected
  arc A29 (-12.035, -3.0434) -> (-13.8108, -5.4875) centre (-4.0724, -10.6959) ccw projected
  arc A30 (-14.6725, -5.2907) -> (-15.2114, -2.3181) centre (-25.7065, -5.7558) ccw projected
  arc A31 (-15.2114, -2.3181) -> (-16.2957, -2.2293) centre (-16.9965, -17.4532) ccw projected
  circle A32 centre (-24.3284, -20.6535) radius 1.6 projected
  circle A33 centre (-13.7961, -24.7851) radius 1.6 projected
  circle A34 centre (-9.6645, -14.2528) radius 1.6 projected
  circle A35 centre (-20.1968, -10.1212) radius 1.6 projected
  line L4 (-7.893, -6.167) -> (-61.9815, 37.4608) projected
  circle A36 centre (8.3767, 1.5633) radius 1.6 projected
  circle A37 centre (-2.3455, -2.0471) radius 1.6 projected
  circle A38 centre (-5.9559, 8.675) radius 1.6 projected
  circle A39 centre (4.7663, 12.2855) radius 1.6 projected
  circle A40 centre (1.2104, 5.1192) radius 2.5 projected
  line L5 (-25.7458, -8.691) -> (-43.1204, -4.145) projected
  line L6 (-44.248, -1.3649) -> (-46.546, 18.0729) projected
  line L7 (-49.1028, -10.0428) -> (-25.2458, -26.6876) projected
  line L8 (-17.326, 27.8341) -> (-20.2818, 28.3476)
  line L9 (-39.7656, 26.479) -> (-40.4462, 33.5769)
  line L10 (-40.4462, 33.5769) -> (-17.6346, 35.7644)
  line L11 (-17.6346, 35.7644) -> (-12.8282, 34.9294)
  line L12 (-9.2052, 11.8155) -> (-17.326, 27.8341)
  line L13 (-20.2818, 28.3476) -> (-39.7656, 26.479)
  line L14 (-12.8282, 34.9294) -> (8.4894, 15.1363)
  circle A41 centre (-16.9965, -17.4532) radius 2 projected
  arc A42 (-13.8108, -5.4875) -> (-14.6725, -5.2907) centre (-16.9965, -17.4532) ccw projected
  arc A43 (5.949, -6.3208) -> (-10.7875, 8.1814) centre (1.2104, 5.1192) ccw projected
  arc A44 (-10.7875, 8.1814) -> (-13.7875, 7.8251) centre (-10.997, -2.8603) ccw projected
  arc A45 (-13.7875, 7.8251) -> (-13.9423, 6.7483) centre (1.2104, 5.1192) ccw projected
  arc A46 (-13.9423, 6.7483) -> (-11.1642, 5.5611) centre (-8.2544, 16.2146) ccw projected
  arc A47 (-11.1642, 5.5611) -> (-11.1642, 4.6772) centre (1.2104, 5.1192) ccw projected
  arc A48 (-11.1642, 4.6772) -> (-13.9423, 3.4901) centre (-8.2544, -5.9763) ccw projected
  arc A49 (-13.9423, 3.4901) -> (-13.7875, 2.4133) centre (1.2104, 5.1192) ccw projected
  arc A50 (-13.7875, 2.4133) -> (-10.7875, 2.0569) centre (-10.997, 13.0986) ccw projected
  arc A51 (-10.7875, 2.0569) -> (-10.5384, 1.2088) centre (1.2104, 5.1192) ccw projected
  arc A52 (-10.5384, 1.2088) -> (-12.8695, -0.7129) centre (-4.7451, -8.1934) ccw projected
  arc A53 (-12.8695, -0.7129) -> (-12.4176, -1.7025) centre (1.2104, 5.1192) ccw projected
  arc A54 (-12.4176, -1.7025) -> (-9.4387, -1.1992) centre (-12.7506, 9.3362) ccw projected
  arc A55 (-9.4387, -1.1992) -> (-8.9608, -1.9429) centre (1.2104, 5.1192) ccw projected
  arc A56 (-8.9608, -1.9429) -> (-10.6561, -4.4435) centre (-0.7533, -9.332) ccw projected
  arc A57 (-10.6561, -4.4435) -> (-9.9437, -5.2656) centre (1.2104, 5.1192) ccw projected
  arc A58 (-9.9437, -5.2656) -> (-7.2273, -3.9435) centre (-13.3732, 5.2321) ccw projected
  arc A59 (-7.2273, -3.9435) -> (-6.5592, -4.5224) centre (1.2104, 5.1192) ccw projected
  arc A60 (-6.5592, -4.5224) -> (-7.4813, -7.3993) centre (3.3977, -9.2999) ccw projected
  arc A61 (-7.4813, -7.3993) -> (-6.5661, -7.9874) centre (1.2104, 5.1192) ccw projected
  arc A62 (-6.5661, -7.9874) -> (-4.3322, -5.9536) centre (-12.8142, 1.1189) ccw projected
  arc A63 (-4.3322, -5.9536) -> (-3.5282, -6.3208) centre (1.2104, 5.1192) ccw projected
  arc A64 (-3.5282, -6.3208) -> (-3.6024, -9.3409) centre (7.3714, -8.0996) ccw projected
  arc A65 (-3.6024, -9.3409) -> (-2.5586, -9.6474) centre (1.2104, 5.1192) ccw projected
  arc A66 (-2.5586, -9.6474) -> (-0.9882, -7.0666) centre (-11.1191, -2.6703) ccw projected
  arc A67 (-0.9882, -7.0666) -> (-0.1132, -7.1924) centre (1.2104, 5.1192) ccw projected
  arc A68 (-0.1132, -7.1924) -> (0.6664, -10.1111) centre (10.846, -5.8284) ccw projected
  arc A69 (0.6664, -10.1111) -> (1.7543, -10.1111) centre (1.2104, 5.1192) ccw projected
  arc A70 (1.7543, -10.1111) -> (2.534, -7.1924) centre (-8.4252, -5.8284) ccw projected
  arc A71 (2.534, -7.1924) -> (3.409, -7.0666) centre (1.2104, 5.1192) ccw projected
  arc A72 (3.409, -7.0666) -> (4.9793, -9.6474) centre (13.5399, -2.6703) ccw projected
  arc A73 (4.9793, -9.6474) -> (6.0232, -9.3409) centre (1.2104, 5.1192) ccw projected
  arc A74 (6.0232, -9.3409) -> (5.949, -6.3208) centre (-4.9506, -8.0996) ccw projected
  circle A75 centre (8.3767, 1.5633) radius 1.6 projected
  circle A76 centre (-2.3455, -2.0471) radius 1.6 projected
  circle A77 centre (-5.9559, 8.675) radius 1.6 projected
  circle A78 centre (4.7663, 12.2855) radius 1.6 projected
  circle A79 centre (1.2104, 5.1192) radius 2.5 projected
  point P0 (0, 0)
  point P1 (8.4894, 15.1363)
  constraints: 14 end point, 8 symmetric about line
extrude "Выдавливание20" add sketch "Эскиз22" against normal up to surface (5 mm away) contours L12 L8 L13 L9 L10 L11 L14 A43
sketch "Эскиз23" plane through (0, 0, 5) normal (0, 0, 1) x (1, 0, 0)
  arc A0 (5.949, -6.3208) -> (8.4894, 15.1363) centre (1.2104, 5.1192) ccw projected
  line L0 (8.4894, 15.1363) -> (-12.8282, 34.9294) projected
  line L1 (-12.8282, 34.9294) -> (-17.6346, 35.7644) projected
  line L2 (-17.6346, 35.7644) -> (-40.4462, 33.5769) projected
  line L3 (-40.4462, 33.5769) -> (-39.7656, 26.479) projected
  line L4 (-39.7656, 26.479) -> (-20.2818, 28.3476) projected
  line L5 (-20.2818, 28.3476) -> (-17.326, 27.8341) projected
  line L6 (-17.326, 27.8341) -> (-9.2052, 11.8155) projected
  arc A1 (-9.2052, 11.8155) -> (-10.7875, 8.1814) centre (1.2104, 5.1192) ccw projected
  arc A2 (-10.7875, 8.1814) -> (-13.7875, 7.8251) centre (-10.997, -2.8603) ccw projected
  arc A3 (-13.7875, 7.8251) -> (-13.9423, 6.7483) centre (1.2104, 5.1192) ccw projected
  arc A4 (-13.9423, 6.7483) -> (-11.1642, 5.5611) centre (-8.2544, 16.2146) ccw projected
  arc A5 (-11.1642, 5.5611) -> (-11.1642, 4.6772) centre (1.2104, 5.1192) ccw projected
  arc A6 (-11.1642, 4.6772) -> (-13.9423, 3.4901) centre (-8.2544, -5.9763) ccw projected
  arc A7 (-13.9423, 3.4901) -> (-13.7875, 2.4133) centre (1.2104, 5.1192) ccw projected
  arc A8 (-13.7875, 2.4133) -> (-10.7875, 2.0569) centre (-10.997, 13.0986) ccw projected
  arc A9 (-10.7875, 2.0569) -> (-10.5384, 1.2088) centre (1.2104, 5.1192) ccw projected
  arc A10 (-10.5384, 1.2088) -> (-12.8695, -0.7129) centre (-4.7451, -8.1934) ccw projected
  arc A11 (-12.8695, -0.7129) -> (-12.4176, -1.7025) centre (1.2104, 5.1192) ccw projected
  arc A12 (-12.4176, -1.7025) -> (-9.4387, -1.1992) centre (-12.7506, 9.3362) ccw projected
  arc A13 (-9.4387, -1.1992) -> (-8.9608, -1.9429) centre (1.2104, 5.1192) ccw projected
  arc A14 (-8.9608, -1.9429) -> (-10.6561, -4.4435) centre (-0.7533, -9.332) ccw projected
  arc A15 (-10.6561, -4.4435) -> (-9.9437, -5.2656) centre (1.2104, 5.1192) ccw projected
  arc A16 (-9.9437, -5.2656) -> (-7.2273, -3.9435) centre (-13.3732, 5.2321) ccw projected
  arc A17 (-7.2273, -3.9435) -> (-6.5592, -4.5224) centre (1.2104, 5.1192) ccw projected
  arc A18 (-6.5592, -4.5224) -> (-7.4813, -7.3993) centre (3.3977, -9.2999) ccw projected
  arc A19 (-7.4813, -7.3993) -> (-6.5661, -7.9874) centre (1.2104, 5.1192) ccw projected
  arc A20 (-6.5661, -7.9874) -> (-4.3322, -5.9536) centre (-12.8142, 1.1189) ccw projected
  arc A21 (-4.3322, -5.9536) -> (-3.5282, -6.3208) centre (1.2104, 5.1192) ccw projected
  arc A22 (-3.5282, -6.3208) -> (-3.6024, -9.3409) centre (7.3714, -8.0996) ccw projected
  arc A23 (-3.6024, -9.3409) -> (-2.5586, -9.6474) centre (1.2104, 5.1192) ccw projected
  arc A24 (-2.5586, -9.6474) -> (-0.9882, -7.0666) centre (-11.1191, -2.6703) ccw projected
  arc A25 (-0.9882, -7.0666) -> (-0.1132, -7.1924) centre (1.2104, 5.1192) ccw projected
  arc A26 (-0.1132, -7.1924) -> (0.6664, -10.1111) centre (10.846, -5.8284) ccw projected
  arc A27 (0.6664, -10.1111) -> (1.7543, -10.1111) centre (1.2104, 5.1192) ccw projected
  arc A28 (1.7543, -10.1111) -> (2.534, -7.1924) centre (-8.4252, -5.8284) ccw projected
  arc A29 (2.534, -7.1924) -> (3.409, -7.0666) centre (1.2104, 5.1192) ccw projected
  arc A30 (3.409, -7.0666) -> (4.9793, -9.6474) centre (13.5399, -2.6703) ccw projected
  arc A31 (4.9793, -9.6474) -> (6.0232, -9.3409) centre (1.2104, 5.1192) ccw projected
  arc A32 (6.0232, -9.3409) -> (5.949, -6.3208) centre (-4.9506, -8.0996) ccw projected
  circle A33 centre (8.3767, 1.5633) radius 1.6 projected
  circle A34 centre (-2.3455, -2.0471) radius 1.6 projected
  circle A35 centre (-5.9559, 8.675) radius 1.6 projected
  circle A36 centre (4.7663, 12.2855) radius 1.6 projected
  circle A37 centre (1.2104, 5.1192) radius 2.5 projected
  arc A38 (9.6552, 14.1752) -> (-10.9233, 7.5887) centre (1.2104, 5.1192) ccw
  arc A39 (-0.5637, -7.1356) -> (3.3993, -7.0683) centre (1.2104, 5.1192) ccw
  arc A40 (3.3993, -7.0683) -> (4.9676, -9.6504) centre (13.5337, -2.6801) ccw
  arc A41 (4.9676, -9.6504) -> (6.0117, -9.3448) centre (1.2104, 5.1192) ccw
  arc A42 (6.0117, -9.3448) -> (5.9399, -6.3245) centre (-4.9611, -8.0947) ccw
  arc A43 (5.9399, -6.3245) -> (6.7442, -5.958) centre (1.2104, 5.1192) ccw
  arc A44 (6.7442, -5.958) -> (8.9765, -7.9936) centre (15.2319, 1.1078) ccw
  arc A45 (8.9765, -7.9936) -> (9.8922, -7.4062) centre (1.2104, 5.1192) ccw
  arc A46 (9.8922, -7.4062) -> (8.9724, -4.5285) centre (-0.9883, -9.2981) ccw
  arc A47 (8.9724, -4.5285) -> (9.6409, -3.9502) centre (1.2104, 5.1192) ccw
  arc A48 (9.6409, -3.9502) -> (12.3562, -5.2745) centre (15.794, 5.2205) ccw
  arc A49 (12.3562, -5.2745) -> (13.0693, -4.4529) centre (1.2104, 5.1192) ccw
  arc A50 (13.0693, -4.4529) -> (11.376, -1.9509) centre (3.1626, -9.3336) ccw
  arc A51 (11.376, -1.9509) -> (11.8545, -1.2077) centre (1.2104, 5.1192) ccw
  arc A52 (11.8545, -1.2077) -> (14.833, -1.7133) centre (15.1747, 9.3251) ccw
  arc A53 (14.833, -1.7133) -> (15.2857, -0.7241) centre (1.2104, 5.1192) ccw
  arc A54 (15.2857, -0.7241) -> (12.9561, 1.1995) centre (7.1553, -8.1981) ccw
  arc A55 (12.9561, 1.1995) -> (13.2058, 2.0474) centre (1.2104, 5.1192) ccw
  arc A56 (13.2058, 2.0474) -> (16.2061, 2.4014) centre (13.4241, 13.089) ccw
  arc A57 (16.2061, 2.4014) -> (16.3618, 3.4781) centre (1.2104, 5.1192) ccw
  arc A58 (16.3618, 3.4781) -> (13.5847, 4.6674) centre (10.6664, -5.9838) ccw
  arc A59 (13.5847, 4.6674) -> (13.5854, 5.5513) centre (1.2104, 5.1192) ccw
  arc A60 (13.5854, 5.5513) -> (16.3644, 6.7362) centre (10.684, 16.2071) ccw
  arc A61 (16.3644, 6.7362) -> (16.2104, 7.8132) centre (1.2104, 5.1192) ccw
  arc A62 (16.2104, 7.8132) -> (13.2107, 8.1719) centre (13.4115, -2.87) ccw
  arc A63 (13.2107, 8.1719) -> (12.9623, 9.0202) centre (1.2104, 5.1192) ccw
  arc A64 (12.9623, 9.0202) -> (15.2949, 10.9401) centre (7.1764, 18.427) ccw
  arc A65 (15.2949, 10.9401) -> (14.8438, 11.93) centre (1.2104, 5.1192) ccw
  arc A66 (14.8438, 11.93) -> (11.8645, 11.4291) centre (15.168, 0.8911) ccw
  arc A67 (11.8645, 11.4291) -> (11.3872, 12.1731) centre (1.2104, 5.1192) ccw
  arc A68 (11.3872, 12.1731) -> (13.0845, 14.6724) centre (3.1855, 19.5688) ccw
  arc A69 (13.0845, 14.6724) -> (12.3727, 15.4951) centre (1.2104, 5.1192) ccw
  arc A70 (12.3727, 15.4951) -> (9.6552, 14.1752) centre (15.7939, 4.9947) ccw
  circle A71 centre (1.4743, 13.1148) radius 1.6
  circle A72 centre (9.206, 4.8553) radius 1.6
  circle A73 centre (0.9465, -2.8765) radius 1.6
  circle A74 centre (-6.7852, 5.3831) radius 1.6
  circle A75 centre (1.2104, 5.1192) radius 2.5
  point P0 (0, 0)
  point P1 (6.3706, 6.1406)
  point P2 (-16.2622, -2.8603)
  point P3 (11.8645, 11.4291)
  point P4 (12.9623, 9.0202)
  point P5 (13.2107, 8.1719)
  point P6 (13.5854, 5.5513)
  point P7 (13.5847, 4.6674)
  point P8 (13.2058, 2.0474)
  point P9 (12.9561, 1.1995)
  point P10 (11.8545, -1.2077)
  point P11 (11.376, -1.9509)
  point P12 (9.6409, -3.9502)
  point P13 (8.9724, -4.5285)
  point P14 (6.7442, -5.958)
  constraints: 66 point on circle, 38 centre point
extrude "Выдавливание21" add sketch "Эскиз23" against normal up to surface (5 mm away) contours A0 A46 A45 A44 | A0 A50 A49 A48 | A0 A54 A53 A52
sketch "Эскиз24" plane through (0, 0, 5) normal (0, 0, 1) x (1, 0, 0)
  arc A0 (5.949, -6.3208) -> (6.7442, -5.958) centre (1.2104, 5.1192) ccw projected
  arc A1 (6.7442, -5.958) -> (8.9765, -7.9936) centre (15.2319, 1.1078) ccw projected
  arc A2 (8.9765, -7.9936) -> (9.8922, -7.4062) centre (1.2104, 5.1192) ccw projected
  arc A3 (9.8922, -7.4062) -> (8.9724, -4.5285) centre (-0.9883, -9.2981) ccw projected
  arc A4 (8.9724, -4.5285) -> (9.6409, -3.9502) centre (1.2104, 5.1192) ccw projected
  arc A5 (9.6409, -3.9502) -> (12.3562, -5.2745) centre (15.794, 5.2205) ccw projected
  arc A6 (12.3562, -5.2745) -> (13.0693, -4.4529) centre (1.2104, 5.1192) ccw projected
  arc A7 (13.0693, -4.4529) -> (11.376, -1.9509) centre (3.1626, -9.3336) ccw projected
  arc A8 (11.376, -1.9509) -> (11.8545, -1.2077) centre (1.2104, 5.1192) ccw projected
  arc A9 (11.8545, -1.2077) -> (14.833, -1.7133) centre (15.1747, 9.3251) ccw projected
  arc A10 (14.833, -1.7133) -> (15.2857, -0.7241) centre (1.2104, 5.1192) ccw projected
  arc A11 (15.2857, -0.7241) -> (12.9561, 1.1995) centre (7.1553, -8.1981) ccw projected
  arc A12 (12.9561, 1.1995) -> (8.4894, 15.1363) centre (1.2104, 5.1192) ccw projected
  line L0 (8.4894, 15.1363) -> (-12.8282, 34.9294) projected
  line L1 (-12.8282, 34.9294) -> (-17.6346, 35.7644) projected
  line L2 (-17.6346, 35.7644) -> (-40.4462, 33.5769) projected
  line L3 (-40.4462, 33.5769) -> (-39.7656, 26.479) projected
  line L4 (-39.7656, 26.479) -> (-20.2818, 28.3476) projected
  line L5 (-20.2818, 28.3476) -> (-17.326, 27.8341) projected
  line L6 (-17.326, 27.8341) -> (-9.2052, 11.8155) projected
  arc A13 (-9.2052, 11.8155) -> (-10.7875, 8.1814) centre (1.2104, 5.1192) ccw projected
  arc A14 (-10.7875, 8.1814) -> (-13.7875, 7.8251) centre (-10.997, -2.8603) ccw projected
  arc A15 (-13.7875, 7.8251) -> (-13.9423, 6.7483) centre (1.2104, 5.1192) ccw projected
  arc A16 (-13.9423, 6.7483) -> (-11.1642, 5.5611) centre (-8.2544, 16.2146) ccw projected
  arc A17 (-11.1642, 5.5611) -> (-11.1642, 4.6772) centre (1.2104, 5.1192) ccw projected
  arc A18 (-11.1642, 4.6772) -> (-13.9423, 3.4901) centre (-8.2544, -5.9763) ccw projected
  arc A19 (-13.9423, 3.4901) -> (-13.7875, 2.4133) centre (1.2104, 5.1192) ccw projected
  arc A20 (-13.7875, 2.4133) -> (-10.7875, 2.0569) centre (-10.997, 13.0986) ccw projected
  arc A21 (-10.7875, 2.0569) -> (-10.5384, 1.2088) centre (1.2104, 5.1192) ccw projected
  arc A22 (-10.5384, 1.2088) -> (-12.8695, -0.7129) centre (-4.7451, -8.1934) ccw projected
  arc A23 (-12.8695, -0.7129) -> (-12.4176, -1.7025) centre (1.2104, 5.1192) ccw projected
  arc A24 (-12.4176, -1.7025) -> (-9.4387, -1.1992) centre (-12.7506, 9.3362) ccw projected
  arc A25 (-9.4387, -1.1992) -> (-8.9608, -1.9429) centre (1.2104, 5.1192) ccw projected
  arc A26 (-8.9608, -1.9429) -> (-10.6561, -4.4435) centre (-0.7533, -9.332) ccw projected
  arc A27 (-10.6561, -4.4435) -> (-9.9437, -5.2656) centre (1.2104, 5.1192) ccw projected
  arc A28 (-9.9437, -5.2656) -> (-7.2273, -3.9435) centre (-13.3732, 5.2321) ccw projected
  arc A29 (-7.2273, -3.9435) -> (-6.5592, -4.5224) centre (1.2104, 5.1192) ccw projected
  arc A30 (-6.5592, -4.5224) -> (-7.4813, -7.3993) centre (3.3977, -9.2999) ccw projected
  arc A31 (-7.4813, -7.3993) -> (-6.5661, -7.9874) centre (1.2104, 5.1192) ccw projected
  arc A32 (-6.5661, -7.9874) -> (-4.3322, -5.9536) centre (-12.8142, 1.1189) ccw projected
  arc A33 (-4.3322, -5.9536) -> (-3.5282, -6.3208) centre (1.2104, 5.1192) ccw projected
  arc A34 (-3.5282, -6.3208) -> (-3.6024, -9.3409) centre (7.3714, -8.0996) ccw projected
  arc A35 (-3.6024, -9.3409) -> (-2.5586, -9.6474) centre (1.2104, 5.1192) ccw projected
  arc A36 (-2.5586, -9.6474) -> (-0.9882, -7.0666) centre (-11.1191, -2.6703) ccw projected
  arc A37 (-0.9882, -7.0666) -> (-0.1132, -7.1924) centre (1.2104, 5.1192) ccw projected
  arc A38 (-0.1132, -7.1924) -> (0.6664, -10.1111) centre (10.846, -5.8284) ccw projected
  arc A39 (0.6664, -10.1111) -> (1.7543, -10.1111) centre (1.2104, 5.1192) ccw projected
  arc A40 (1.7543, -10.1111) -> (2.534, -7.1924) centre (-8.4252, -5.8284) ccw projected
  arc A41 (2.534, -7.1924) -> (3.409, -7.0666) centre (1.2104, 5.1192) ccw projected
  arc A42 (3.409, -7.0666) -> (4.9793, -9.6474) centre (13.5399, -2.6703) ccw projected
  arc A43 (4.9793, -9.6474) -> (6.0232, -9.3409) centre (1.2104, 5.1192) ccw projected
  arc A44 (6.0232, -9.3409) -> (5.949, -6.3208) centre (-4.9506, -8.0996) ccw projected
  circle A45 centre (8.3767, 1.5633) radius 1.6 projected
  circle A46 centre (-2.3455, -2.0471) radius 1.6 projected
  circle A47 centre (-5.9559, 8.675) radius 1.6 projected
  circle A48 centre (4.7663, 12.2855) radius 1.6 projected
  circle A49 centre (1.2104, 5.1192) radius 2.5 projected
  line L7 (-17.35, 43.8487) -> (-22.1564, 44.6837)
  line L8 (-22.1564, 44.6837) -> (-44.9679, 42.4962)
  line L9 (-44.9679, 42.4962) -> (-44.2873, 35.3983)
  line L10 (-44.2873, 35.3983) -> (-24.8035, 37.2669)
  line L11 (-24.8035, 37.2669) -> (-21.8477, 36.7534)
  line L12 (-17.326, 27.8341) -> (-21.8477, 36.7534)
  line L13 (-17.326, 27.8341) -> (-9.2052, 11.8155) projected
  line L14 (-12.8282, 34.9294) -> (-35.5945, 56.0675)
  line L15 (8.4894, 15.1363) -> (-12.8282, 34.9294) projected
  line L16 (-36.7753, 48.5005) -> (0.9516, 41.946)
  line L17 (-17.326, 27.8341) -> (-12.8282, 34.9294)
  line L18 (-21.8477, 36.7534) -> (-15.7767, 46.3305)
  line L19 (-17.35, 43.8487) -> (8.4894, 15.1363)
  point P0 (0, 0)
  dimension "d79" = 10
  constraints: 22 end point, 2 collinear, 2 parallel, 1 point on line
  measures "d79" distance of L5.end L12.end
extrude "Выдавливание22" add sketch "Эскиз24" against normal up to surface (5 mm away) contours L0 L14 L18 L19 | L17 L12 L2 L1 | L1 L2 L12 L18 L14 | L18 L14 L8 L7 | L18 L11 L10 L9 L8 L14